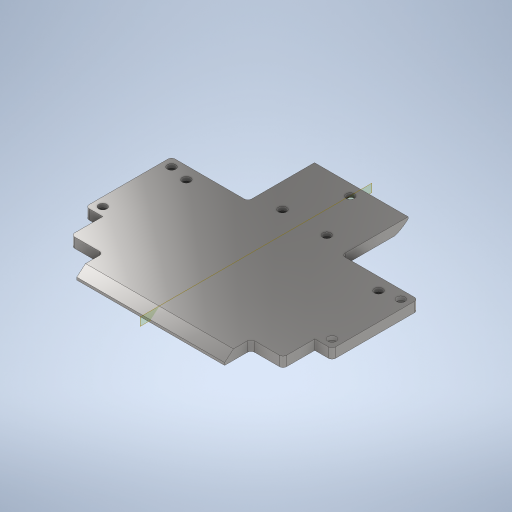
# Autodesk Inventor part: podstawa
Saved by Autodesk Inventor 2023 (Build 270158000, 158)
## iProperties
Created: 2025-01-11
Part Number: podstawa
Material: Stal, odlew
Document SubType Name: Modeling
Designer: kamil
Density: 7.85 g/cm^3
Appearance: Częściowo polerowany
Mass: 185.986 g
Surface Area: 141.567 cm^2
Volume: 23.6924 cm^3
Author: kamil
Autodesk Inventor part; units mm, degrees
ref_plane "YZ Plane" through (0, 0, 0) normal (1, 0, 0) x (0, 1, 0)
ref_plane "XZ Plane" through (0, 0, 0) normal (0, 1, 0) x (-1, 0, 0)
ref_plane "XY Plane" through (0, 0, 0) normal (0, 0, 1) x (1, 0, 0)
sketch "Szkic1" plane through (0, 0, 0) normal (0, 1, 0) x (-1, 0, 0)
  line L0 (50, 50) -> (-50, 50)
  line L1 (-50, 50) -> (-50, -50)
  line L2 (-50, -50) -> (50, -50)
  line L3 (50, -50) -> (50, 50)
  line L4 (50, 50) -> (-50, -50) construction
  line L5 (-50, 50) -> (50, -50) construction
  point P0 (0, 0)
  dimension "d0" = 100
  dimension "d1" = 100
  constraints: 12 end point, 2 midpoint, 2 parallel, 1 horizontal, 1 perpendicular
  measures "d0" distance of L2.end L1.end
  measures "d1" distance of L1.end L0.end
extrude "Wyciągnięcie proste1" add sketch "Szkic1" along normal blind 3
sketch "Szkic2" plane through (0, 3, 0) normal (0, 1, 0) x (1, 0, 0)
  line L0 (50, -50) -> (50, 50) projected
  line L1 (50, 50) -> (-50, 50) projected
  line L2 (-50, 50) -> (-50, -50) projected
  line L3 (-50, -50) -> (50, -50) projected
  line L4 (-50, 50) -> (-19, 50)
  line L5 (-19, 50) -> (-19, 17)
  line L6 (-19, 17) -> (-50, 17)
  line L7 (-50, 17) -> (-50, 50)
  line L8 (50, 50) -> (19, 50)
  line L9 (19, 50) -> (19, 17)
  line L10 (19, 17) -> (50, 17)
  line L11 (50, 17) -> (50, 50)
  point P0 (0, 0)
  dimension "d4" = 31
  dimension "d5" = 33
  dimension "d6" = 31
  constraints: 16 end point, 4 parallel, 2 horizontal, 2 perpendicular, 1 horizontal alignment
  measures "d4" distance of L5.end L6.end
  measures "d5" distance of L4.end L5.end
  measures "d6" distance of L10.end L9.end
extrude "Wyciągnięcie proste2" cut sketch "Szkic2" against normal through all contours L10 L9 L1 L0 | L2 L1 L5 L6
sketch "Szkic3" plane through (0, 3, 0) normal (0, 1, 0) x (1, 0, 0)
  line L0 (19, 17) -> (19, 50) projected
  line L1 (19, 50) -> (-19, 50) projected
  line L2 (-19, 50) -> (-19, 17) projected
  line L3 (-19, 17) -> (-50, 17) projected
  line L4 (-50, 17) -> (-50, -50) projected
  line L5 (-50, -50) -> (50, -50) projected
  line L6 (50, -50) -> (50, 17) projected
  line L7 (50, 17) -> (19, 17) projected
  line L8 (19, 50) -> (-19, 50)
  line L9 (-19, 50) -> (-19, 44)
  line L10 (-19, 44) -> (19, 44)
  line L11 (19, 44) -> (19, 50)
  point P0 (0, 0)
  dimension "d9" = 6
  constraints: 8 end point, 2 parallel, 1 horizontal, 1 perpendicular, 1 point on line
  measures "d9" distance of L9.end L8.end
extrude "Wyciągnięcie proste3" cut sketch "Szkic3" against normal through all contours L10 L2 L1 L0
sketch "Szkic5" plane through (-50, 0, 50) normal (-1, 0, 0) x (0, 0, 1)
  line L0 (0, 0) -> (0, 3) projected
  line L1 (-67, 3) -> (-67, 0) projected
  line L2 (-67, 0) -> (0, 0) projected
  line L3 (0, 0) -> (0, 3) projected
  line L4 (-67, 3) -> (0, 3) projected
  line L5 (-4.6672, -3.25) -> (-21.0795, 10.5216) projected
  point P0 (-50, 0)
  point P1 (-12.1156, 3)
  point P2 (-8.5404, 0)
extrude "Wyciągnięcie proste5" cut sketch "Szkic5" against normal through all contours L2 L5 L4 L0
sketch "Szkic6" plane through (0, 0, 0) normal (0, -1, 0) x (1, 0, 0)
  line L0 (-50, 17.8844) -> (-43, 17.8844) projected
  line L1 (-50, 17.8844) -> (-43, 17.8844)
  line L2 (-43, 17.8844) -> (-43, 43.0531)
  line L3 (-43, 43.0531) -> (-50, 43.0531)
  line L4 (-50, 43.0531) -> (-50, 17.8844)
  point P0 (0, 0)
  constraints: 8 end point, 2 parallel, 1 horizontal, 1 perpendicular
extrude "Wyciągnięcie proste6" cut sketch "Szkic6" against normal through all
ref_plane "Płaszczyzna konstrukcyjna1" through (0, 0, -17) normal (-1, 0, 0) x (0, 0, 1)
mirror "Odbij1" about plane through (0, 0, -17) normal (-1, 0, 0) of "Wyciągnięcie proste6"
sketch "Szkic8" plane through (0, 0, 0) normal (0, -1, 0) x (1, 0, 0)
  line L0 (50, 17.8844) -> (43, 17.8844) projected
  line L1 (43, 17.8844) -> (43, 41.4596) projected
  line L2 (43, 41.4596) -> (-43, 41.4596) projected
  line L3 (-43, 41.4596) -> (-43, 17.8844) projected
  line L4 (-43, 17.8844) -> (-50, 17.8844) projected
  line L5 (-50, -17) -> (-50, 17.8844) projected
  line L6 (-50, -17) -> (-19, -17) projected
  line L7 (-19, -17) -> (-19, -44) projected
  line L8 (-19, -44) -> (19, -44) projected
  line L9 (19, -44) -> (19, -17) projected
  line L10 (19, -17) -> (50, -17) projected
  line L11 (50, 17.8844) -> (50, -17) projected
  point P0 (0, 0)
extrude "Wyciągnięcie proste7" add sketch "Szkic8" along normal blind 1
sketch "Szkic9" plane through (-19, 3, -44) normal (-1, 0, 0) x (0, 0, 1)
  circle A0 centre (10, 9.75) radius 16 projected
  circle A1 centre (10, 9.75) radius 14.5
  line L0 (0, 0) -> (0, -4) projected
  line L1 (27, -4) -> (0, -4) projected
  line L2 (27, 0) -> (27, -4) projected
  line L3 (0, 0) -> (27, 0) projected
  point P0 (44, -3)
  point P1 (5.397, -4)
  point P2 (0, -0.75)
  dimension "d21" = 1.5
  constraints: 1 centre point
  measures "d21" radial gap between concentric circles of A0 A1
extrude "Wyciągnięcie proste8" cut sketch "Szkic9" against normal through all contours L0 A1 L1 A0 | A0 L1 L0
sketch "Szkic10" plane through (0, -1, 0) normal (0, -1, 0) x (1, 0, 0)
  point P0 (0, 0)
sketch "Szkic11" plane through (0, -1, 0) normal (0, -1, 0) x (1, 0, 0)
  circle A0 centre (0, -39.5) radius 1.7 projected
  circle A1 centre (-9, -21) radius 1.7 projected
  circle A2 centre (9, -21) radius 1.7 projected
  arc A3 (46.5, -10) -> (43, -13.5) centre (46.5, -13.5) ccw projected
  arc A4 (43, 14.3844) -> (47, 10.9203) centre (46.5, 14.3844) ccw projected
  arc A5 (-43, -13.5) -> (-46.5, -10) centre (-46.5, -13.5) ccw projected
  arc A6 (-47, 10.9203) -> (-43, 14.3844) centre (-46.5, 14.3844) ccw projected
  circle A7 centre (-39, -12) radius 1.55 projected
  circle A8 centre (39, -12) radius 1.55 projected
  point P0 (0, 0)
hole "Otwór1" at (-39, -1, -12) at (-46.5, -1, -13.5) at (-46.5, -1, 14.3844) at (-9, -1, -21) at (0, -1, -39.5) at (9, -1, -21) at (39, -1, -12) at (46.5, -1, -13.5) at (46.5, -1, 14.3844) direction (0, 1, 0) diameter 3.3 end through all counterbore diameter 6.2 counterbore depth 2.4
sketch "Szkic12" plane through (0, -1, 0) normal (0, -1, 0) x (1, 0, 0)
  arc A0 (2.9674, -38.603) -> (-2.9674, -38.603) centre (0, -39.5) ccw projected
  line L0 (2.9674, -38.603) -> (19, -38.603) projected
  line L1 (19, -38.603) -> (19, -17) projected
  line L2 (19, -17) -> (50, -17) projected
  line L3 (50, -17) -> (50, 17.8844) projected
  line L4 (50, 17.8844) -> (43, 17.8844) projected
  line L5 (43, 17.8844) -> (43, 41.4596) projected
  line L6 (43, 41.4596) -> (-43, 41.4596) projected
  line L7 (-43, 41.4596) -> (-43, 17.8844) projected
  line L8 (-43, 17.8844) -> (-50, 17.8844) projected
  line L9 (-50, 17.8844) -> (-50, -17) projected
  line L10 (-50, -17) -> (-19, -17) projected
  line L11 (-19, -17) -> (-19, -38.603) projected
  line L12 (-19, -38.603) -> (-2.9674, -38.603) projected
  circle A1 centre (46.5, 14.3844) radius 3.1 projected
  circle A2 centre (39, -12) radius 3.1 projected
  circle A3 centre (-46.5, 14.3844) radius 3.1 projected
  circle A4 centre (-39, -12) radius 3.1 projected
  circle A5 centre (-46.5, -13.5) radius 3.1 projected
  circle A6 centre (-9, -21) radius 3.1 projected
  circle A7 centre (9, -21) radius 3.1 projected
  circle A8 centre (46.5, -13.5) radius 3.1 projected
  line L13 (-50, 30.7663) -> (-50, 40.7446) projected
  line L14 (-43, 30.7663) -> (-50, 30.7663) projected
  line L15 (-43, 40.7446) -> (-43, 30.7663) projected
  line L16 (-43, 40.7446) -> (-50, 40.7446) projected
  line L17 (-50, 30.7663) -> (-30, 30.7663)
  line L18 (-30, 30.7663) -> (-30, 41.4596)
  line L19 (-30, 41.4596) -> (-50, 41.4596)
  line L20 (-50, 41.4596) -> (-50, 30.7663)
  line L21 (50, 30.7663) -> (50, 40.7446) projected
  line L22 (43, 40.7446) -> (50, 40.7446) projected
  line L23 (43, 40.7446) -> (43, 30.7663) projected
  line L24 (43, 30.7663) -> (50, 30.7663) projected
  line L25 (50, 30.7663) -> (30, 30.7663)
  line L26 (30, 30.7663) -> (30, 41.4596)
  line L27 (30, 41.4596) -> (50, 41.4596)
  line L28 (50, 41.4596) -> (50, 30.7663)
  circle A9 centre (46.1444, 33.7663) radius 1.1 projected
  circle A10 centre (-46.1444, 33.7663) radius 1.1 projected
  point P0 (0, 0)
  dimension "d31" = 20
  dimension "d32" = 20
  constraints: 16 end point, 4 parallel, 2 horizontal, 2 perpendicular, 2 point on line
  measures "d31" distance of L19.end L18.end
  measures "d32" distance of L26.end L27.end
extrude "Wyciągnięcie proste9" cut sketch "Szkic12" against normal through all contours L25 L26 L6 L5 | L5 L22 L21 L24 | L14 L13 L16 L7 | L7 L6 L18 L17 | L5 L27 L28 L22 | L16 L20 L19 L7 | A9 | A10
fillet "Zaokrąglenie2" radius 1.5 10 edges at (-50, 1, 17.8844) (-50, 1, -17) (-19, 1, -17) (19, 1, -17) (50, 1, -17) (50, 1, 17.8844) (43, 1, 30.7663) (30, 1, 30.7663) (-43, 1, 30.7663) (-30, 1, 30.7663)
